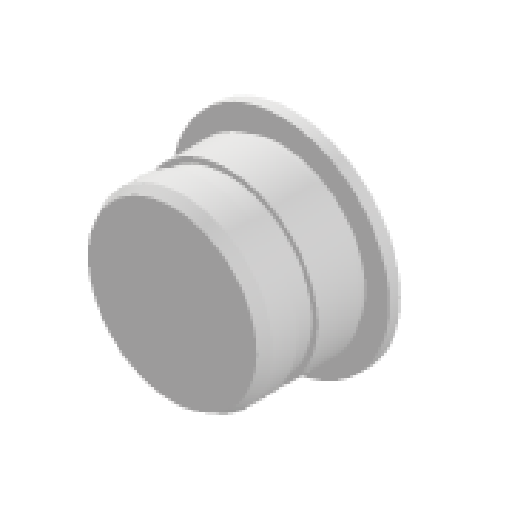
# Autodesk Inventor part: Моторчик_Замка
Saved by Autodesk Inventor 2026 (Build 300175000, 175)
## iProperties
Created: 2026-04-20
Part Number: Моторчик_Замка
Material: Типовые
Document SubType Name: Modeling
Designer: Artem Sannikov
Density: 1 g/cm^3
Appearance: По умолчанию
Author: Artem Sannikov
Autodesk Inventor part; units mm, degrees
ref_plane "YZ Plane" through (0, 0, 0) normal (1, 0, 0) x (0, 1, 0)
ref_plane "XZ Plane" through (0, 0, 0) normal (0, 1, 0) x (-1, 0, 0)
ref_plane "XY Plane" through (0, 0, 0) normal (0, 0, 1) x (1, 0, 0)
sketch "Эскиз1" plane through (0, 0, 0) normal (1, 0, 0) x (0, 1, 0)
  line L0 (-2.4368, -6.5267) -> (-2.4368, 6.8727)
  line L1 (-2.4368, 6.8727) -> (-30.6461, 6.8727)
  line L2 (-30.6461, 6.8727) -> (-30.6461, 10.1168)
  line L3 (-30.6461, 10.1168) -> (-23.8759, 10.1168)
  line L4 (-23.8759, 10.1168) -> (-23.8759, 12.7967)
  line L5 (-23.8759, 12.7967) -> (-25.4274, 12.7967)
  line L6 (-25.4274, 12.7967) -> (-25.4274, 25.2088)
  line L7 (-25.4274, 25.2088) -> (-23.8759, 25.2088)
  line L8 (-23.8759, 25.2088) -> (-23.8759, 30.8506)
  line L9 (-23.8759, 30.8506) -> (-25.4274, 30.8506)
  line L10 (-25.4274, 30.8506) -> (-25.4274, 37.903)
  line L11 (-25.4274, 37.903) -> (-23.8759, 40.8649)
  line L12 (-23.8759, 40.8649) -> (0, 40.8649)
  line L13 (0, 40.8649) -> (0, -6.5267)
  line L14 (0, -6.5267) -> (-2.4368, -6.5267)
  point P0 (0, 0)
  constraints: 30 end point, 10 perpendicular, 5 point on line, 1 parallel, 1 vertical
revolve "Вращение1" add sketch "Эскиз1" angle 360 about axis through (0, 0, 40.8649) along (0, 0, -1)
